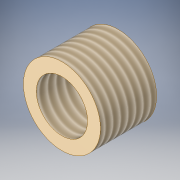
# Autodesk Inventor part: Part8
Saved by Autodesk Inventor 2019.1 (Build 231200000, 200)
## iProperties
Created: 2018-09-18
Part Number: Part8
Material: Polyethylene, High Density
Document SubType Name: Modeling
Designer: drawing
Density: 0.952 g/cm^3
Appearance: Smooth - Off-White
Author: drawing
Autodesk Inventor part; units mm, degrees
ref_plane "YZ Plane" through (0, 0, 0) normal (1, 0, 0) x (0, 1, 0)
ref_plane "XZ Plane" through (0, 0, 0) normal (0, 1, 0) x (-1, 0, 0)
ref_plane "XY Plane" through (0, 0, 0) normal (0, 0, 1) x (1, 0, 0)
sketch "Sketch1" plane through (0, 0, 0) normal (0, 0, 1) x (1, 0, 0)
  circle A0 centre (0, 0) radius 7.1437
  circle A1 centre (0, 0) radius 4.7625
  dimension "d0" = 14.2875
  dimension "d1" = 9.525
  constraints: 2 centre point, 2 coincident
  measures "d0" diameter of A0
  measures "d1" diameter of A1
extrude "Extrusion1" add sketch "Sketch1" along normal blind 10.414
thread "Thread1" size "9/16-18 UNF" class "2A" standard "ANSI Unified Screw Threads" full length
thread "Thread2" size "3/8-16 UNC" class "2B" standard "ANSI Unified Screw Threads" full length
body "Solid1"
